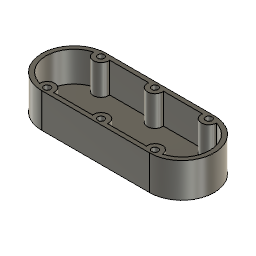
robosoc_motor_case_noHole (Autodesk Fusion 360 design; units mm, degrees)
part number: 2025-12-10-15-49-31-313
Autodesk Fusion 360 part; units mm, degrees
sketch "Sketch1" plane through (0, 0, 0) normal (0, 0, 1) x (1, 0, 0)
  line L0 (15, 0) -> (65, 0)
  line L1 (65, 30) -> (15, 30)
  arc A0 (15, 30) -> (0, 15) centre (15, 15) ccw
  arc A1 (0, 15) -> (15, 0) centre (15, 15) ccw
  arc A2 (80, 15) -> (65, 30) centre (65, 15) ccw
  arc A3 (65, 0) -> (80, 15) centre (65, 15) ccw
  line L2 (15, 15) -> (65, 15) construction
  line L3 (15, 15) -> (15, 27.5) construction
  line L4 (65, 15) -> (65, 27.5) construction
  line L5 (15, 27.5) -> (40, 27.5) construction
  circle A4 centre (15, 27.5) radius 1.5
  circle A5 centre (40, 27.5) radius 1.5
  circle A6 centre (65, 27.5) radius 1.5
  circle A7 centre (15, 2.5) radius 1.5
  circle A8 centre (40, 2.5) radius 1.5
  circle A9 centre (65, 2.5) radius 1.5
  circle A10 centre (65, 15) radius 2.5
  circle A11 centre (15, 15) radius 2.5
  point P0 (80, 0)
  point P1 (0, 30)
  dimension "d1" = 80
  dimension "d2" = 30
  dimension "d3" = 15
  dimension "d4" = 15
  dimension "d5" = 15
  dimension "d6" = 15
  dimension "d7" = 12.5
  dimension "d8" = 12.5
  dimension "d9" = 25
  dimension "d11" = 3
  dimension "d12" = 3
  dimension "d13" = 3
  dimension "d22" = 5
  dimension "d23" = 5
  constraint horizontal L0
  constraint horizontal L1
  constraint coincident P1 L1
  constraint tangent L1 A0
  constraint coincident origin L0
  constraint tangent L0 A1
  constraint coincident A0.end A1.start
  constraint tangent L1 A2
  constraint coincident P0 L0
  constraint tangent L0 A3
  constraint coincident A2.start A3.end
  constraint coincident A0.centre A1.centre
  constraint coincident A2.centre A3.centre
  constraint perpendicular L1 L3
  constraint perpendicular L2 L4
  constraint perpendicular L3 L5
  constraint coincident L3.end L5.start
  constraint coincident L5.end A5.centre
  constraint coincident L4.end A6.centre
  constraint symmetric L2 A4 A7
  constraint symmetric L2 A5 A8
  constraint symmetric L2 A6 A9
  constraint concentric A3 A10
  constraint concentric A1 A11
  measures "d1" distance of origin P0
  measures "d2" distance of origin P1
  measures "d3" radius of A0
  measures "d4" radius of A1
  measures "d5" radius of A2
  measures "d6" radius of A3
  measures "d7" distance of A0.centre L3.end
  measures "d8" distance of A2.centre L4.end
  measures "d9" distance of L3.end L5.end
  measures "d11" diameter of A4
  measures "d12" diameter of A5
  measures "d13" diameter of A6
  measures "d22" diameter of A10
  measures "d23" diameter of A11
extrude "Extrude1" add sketch "Sketch1" along normal blind 16 contours L0 L1 A0 A1 A2 A3 | A10 | A11
shell "Shell1" thickness 2 removed faces 1 at (23.6999, 18.8266, 16)
hole "Hole1" at (65, 27.5, 0) at (40, 27.5, 0) at (15, 27.5, 0) at (15, 2.5, 0) at (40, 2.5, 0) at (65, 2.5, 0) direction (0, 0, 1) diameter 4 depth 1 tip angle 180 countersink diameter 4.4 countersink angle 90
extrude "Extrude2" add sketch "Sketch1" against normal blind 4 draft -15 contours A10 | A11
equation "d23 = d22"
